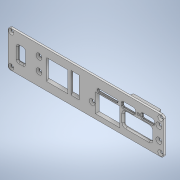
# Autodesk Inventor part: back_panel
Saved by Autodesk Inventor 2021 (Build 250183000, 183)
## iProperties
Created: 2026-03-01
Part Number: back_panel
Material: Generic
Document SubType Name: Modeling
Designer: Toby
Density: 1 g/cm^3
Appearance: Default
Author: Toby
Autodesk Inventor part; units mm, degrees
ref_plane "YZ Plane" through (0, 0, 0) normal (1, 0, 0) x (0, 1, 0)
ref_plane "XZ Plane" through (0, 0, 0) normal (0, 1, 0) x (-1, 0, 0)
ref_plane "XY Plane" through (0, 0, 0) normal (0, 0, 1) x (1, 0, 0)
sketch "Sketch1" plane through (0, 0, 0) normal (0, 0, 1) x (1, 0, 0)
  line L0 (-59.9, 14.1) -> (60.3, 14.1)
  line L1 (60.3, 14.1) -> (60.3, -14.1)
  line L2 (60.3, -14.1) -> (-59.9, -14.1)
  line L3 (-59.9, -14.1) -> (-59.9, 14.1)
  point P0 (0, 0)
  dimension "d0" = 120.2
  dimension "d1" = 28.2
  dimension "d2" = 59.9
  dimension "d3" = 14.1
  constraints: 8 end point, 2 parallel, 1 horizontal, 1 perpendicular
  measures "d0" distance of L0.start L0.end
  measures "d1" distance of L2.end L0.start
  measures "d2" distance from line of point (0, 0) L3
  measures "d3" distance from line of point (0, 0) L0
extrude "Extrusion1" add sketch "Sketch1" along normal blind 1.5
fillet "Fillet1" radius 2 4 edges at (-59.9, 14.1, 0.75) (60.3, 14.1, 0.75) (60.3, -14.1, 0.75) (-59.9, -14.1, 0.75)
sketch "Sketch2" plane through (0, 0, 1.5) normal (0, 0, 1) x (1, 0, 0)
  line L0 (-59.9, 12.1) -> (-59.9, -12.1) projected
  line L1 (58.3, 14.1) -> (-57.9, 14.1) projected
  line L2 (-57.9, -14.1) -> (58.3, -14.1) projected
  line L3 (60.3, -12.1) -> (60.3, 12.1) projected
  point P0 (0, 0)
  point P1 (-57.5, 11.7)
  point P2 (-57.5, -11.7)
  point P3 (57.9, 11.7)
  point P4 (57.9, -11.7)
  dimension "d7" = 2.4
  dimension "d8" = 2.4
  dimension "d9" = 2.4
  dimension "d10" = 2.4
  dimension "d11" = 2.4
  dimension "d12" = 2.4
  dimension "d13" = 2.4
  dimension "d14" = 2.4
  measures "d7" distance from line of L0 point (-57.5, 11.7)
  measures "d8" distance from line of L1 point (-57.5, 11.7)
  measures "d9" distance from line of L2 point (-57.5, -11.7)
  measures "d10" distance from line of L0 point (-57.5, -11.7)
  measures "d11" distance from line of L1 point (57.9, 11.7)
  measures "d12" distance from line of L3 point (57.9, 11.7)
  measures "d13" distance from line of L2 point (57.9, -11.7)
  measures "d14" distance from line of L3 point (57.9, -11.7)
hole "Hole1" at (-57.5, 11.7, 1.5) at (-57.5, -11.7, 1.5) at (57.9, 11.7, 1.5) at (57.9, -11.7, 1.5) direction (0, 0, -1) diameter 2 depth 4 tip angle 118 countersink diameter 4 countersink angle 90
sketch "Sketch3" plane through (0, 0, 1.5) normal (0, 0, 1) x (1, 0, 0)
  circle A0 centre (-57.5, -11.7) radius 1 projected
  circle A1 centre (-57.5, 11.7) radius 1 projected
  line L0 (-55.9, 14.1) -> (60.3, 14.1)
  line L1 (60.3, 14.1) -> (60.3, -14)
  line L2 (60.3, -14) -> (-55.9, -14)
  line L3 (-55.9, -14) -> (-55.9, 14.1)
  line L4 (-59.9, 12.1) -> (-59.9, -12.1) projected
  line L5 (-57.9, -14.1) -> (58.3, -14.1) projected
  line L6 (58.3, 14.1) -> (-57.9, 14.1) projected
  line L7 (60.3, -12.1) -> (60.3, 12.1) projected
  line L8 (-52.5, 5.1) -> (-47.3, 5.1)
  line L9 (-47.3, 5.1) -> (-47.3, -5.6)
  line L10 (-47.3, -5.6) -> (-52.5, -5.6)
  line L11 (-52.5, -5.6) -> (-52.5, 5.1)
  circle A2 centre (-35.9, 6) radius 1
  circle A3 centre (-35.9, -4) radius 1
  circle A4 centre (5.1, -4) radius 1
  circle A5 centre (56.6, -4) radius 1
  circle A6 centre (56.6, 6) radius 1
  line L12 (-30, 6.7) -> (-13.7, 6.7)
  line L13 (-13.7, 6.7) -> (-13.7, -6.3)
  line L14 (-13.7, -6.3) -> (-30, -6.3)
  line L15 (-30, -6.3) -> (-30, 6.7)
  line L16 (9.1, 4) -> (25.1, 4)
  line L17 (25.1, 4) -> (25.1, -9)
  line L18 (25.1, -9) -> (9.1, -9)
  line L19 (9.1, -9) -> (9.1, 4)
  line L20 (29.1, 2) -> (51.1, 2)
  line L21 (51.1, 2) -> (51.1, -8)
  line L22 (51.1, -8) -> (29.1, -8)
  line L23 (29.1, -8) -> (29.1, 2)
  line L24 (28.1, 7.9) -> (38, 7.9)
  line L25 (38, 7.9) -> (38, 4.2)
  line L26 (38, 4.2) -> (28.1, 4.2)
  line L27 (28.1, 4.2) -> (28.1, 7.9)
  line L28 (43.3, 7.9) -> (52.8, 7.9)
  line L29 (52.8, 7.9) -> (52.8, 4.2)
  line L30 (52.8, 4.2) -> (43.3, 4.2)
  line L31 (43.3, 4.2) -> (43.3, 7.9)
  line L32 (-11.2, 7.5) -> (-4.9, 7.5)
  line L33 (-4.9, 7.5) -> (-4.9, -6)
  line L34 (-4.9, -6) -> (-11.2, -6)
  line L35 (-11.2, -6) -> (-11.2, 7.5)
  line L36 (9.1, 5) -> (25.1, 5)
  line L37 (25.1, 5) -> (25.1, 7.5)
  line L38 (25.1, 7.5) -> (9.1, 7.5)
  line L39 (9.1, 7.5) -> (9.1, 5)
  point P0 (0, 0)
  dimension "d22" = 23.4
  dimension "d23" = 4
  dimension "d24" = 0.1
  dimension "d25" = 8.4
  dimension "d26" = 19.1
  dimension "d27" = 3.4
  dimension "d28" = 8.6
  dimension "d31" = 2
  dimension "d32" = 2
  dimension "d35" = 10
  dimension "d36" = 10
  dimension "d37" = 2
  dimension "d38" = 61
  dimension "d39" = 10
  dimension "d40" = 2
  dimension "d41" = 2
  dimension "d42" = 112.5
  dimension "d43" = 112.5
  dimension "d45" = 20
  dimension "d46" = 10
  dimension "d47" = 25.9
  dimension "d48" = 42.2
  dimension "d49" = 7.7
  dimension "d50" = 20.7
  dimension "d51" = 44.7
  dimension "d52" = 51
  dimension "d53" = 21.5
  dimension "d54" = 8
  dimension "d55" = 65
  dimension "d56" = 81
  dimension "d57" = 85
  dimension "d58" = 107
  dimension "d59" = 5
  dimension "d60" = 18
  dimension "d61" = 6
  dimension "d62" = 16
  dimension "d63" = 2.5
  dimension "d64" = 1
  dimension "d65" = 84
  dimension "d66" = 93.9
  dimension "d67" = 99.2
  dimension "d68" = 108.7
  dimension "d69" = 18.2
  dimension "d70" = 22
  dimension "d104" = 20
  dimension "d105" = 20
  constraints: 72 end point, 18 parallel, 9 horizontal, 9 perpendicular, 5 centre point, 4 collinear, 2 point on line
  measures "d22" distance of A0.centre A1.centre
  measures "d23" distance between parallel lines of L4 L3
  measures "d24" distance between parallel lines of L5 L2
  measures "d25" distance between parallel lines of L2 L10
  measures "d26" distance between parallel lines of L2 L8
  measures "d27" distance between parallel lines of L3 L11
  measures "d28" distance between parallel lines of L3 L9
  measures "d31" diameter of A2
  measures "d32" diameter of A3
  measures "d35" distance from line of A3.centre L2
  measures "d36" distance of A3.centre A2.centre
  measures "d37" diameter of A4
  measures "d38" distance from line of L3 A4.centre
  measures "d39" distance from line of L2 A4.centre
  measures "d40" diameter of A5
  measures "d41" diameter of A6
  measures "d42" distance from line of L3 A5.centre
  measures "d43" distance from line of L3 A6.centre
  measures "d45" distance from line of L2 A6.centre
  measures "d46" distance from line of L2 A5.centre
  measures "d47" distance between parallel lines of L3 L15
  measures "d48" distance between parallel lines of L3 L13
  measures "d49" distance between parallel lines of L2 L14
  measures "d50" distance between parallel lines of L2 L12
  measures "d51" distance between parallel lines of L3 L35
  measures "d52" distance between parallel lines of L3 L33
  measures "d53" distance between parallel lines of L2 L32
  measures "d54" distance between parallel lines of L2 L34
  measures "d55" distance between parallel lines of L3 L19
  measures "d56" distance between parallel lines of L3 L17
  measures "d57" distance between parallel lines of L3 L23
  measures "d58" distance between parallel lines of L3 L21
  measures "d59" distance between parallel lines of L2 L18
  measures "d60" distance between parallel lines of L2 L16
  measures "d61" distance between parallel lines of L2 L22
  measures "d62" distance between parallel lines of L2 L20
  measures "d63" distance between parallel lines of L36 L38
  measures "d64" distance between parallel lines of L16 L36
  measures "d65" distance between parallel lines of L3 L27
  measures "d66" distance between parallel lines of L3 L25
  measures "d67" distance between parallel lines of L3 L31
  measures "d68" distance between parallel lines of L3 L29
  measures "d69" distance between parallel lines of L2 L26
  measures "d70" distance between parallel lines of L5 L24
  measures "d104" distance from line of L3 A2.centre
  measures "d105" distance from line of L3 A3.centre
extrude "Extrusion2" cut sketch "Sketch3" against normal blind 1.5 contours L8 L9 L10 L11 | A2 | A3 | A4 | A5 | A6 | L12 L13 L14 L15 | L16 L17 L18 L19 | L20 L21 L22 L23 | L24 L25 L26 L27 | L28 L29 L30 L31 | L32 L33 L34 L35 | L39 L38 L37 L36
fillet "Fillet3" radius 1 8 edges at (28.1, 7.9, 0.75) (28.1, 4.2, 0.75) (38, 7.9, 0.75) (38, 4.2, 0.75) (43.3, 7.9, 0.75) (43.3, 4.2, 0.75) (52.8, 7.9, 0.75) (52.8, 4.2, 0.75)
fillet "Fillet4" radius 2 4 edges at (29.1, 2, 0.75) (29.1, -8, 0.75) (51.1, -8, 0.75) (51.1, 2, 0.75)
chamfer "Chamfer1" distance 1 angle 45 8 edges at (40.1, 2, 1.5) (50.5142, 1.4142, 1.5) (51.1, -3, 1.5) (50.5142, -7.4142, 1.5) (40.1, -8, 1.5) (29.6858, -7.4142, 1.5) (29.1, -3, 1.5) (29.6858, 1.4142, 1.5)
fillet "Fillet5" radius 1 4 edges at (-52.5, 5.1, 0.75) (-47.3, 5.1, 0.75) (-52.5, -5.6, 0.75) (-47.3, -5.6, 0.75)
chamfer "Chamfer2" distance 0.6 angle 45 16 edges at (33.05, 7.9, 1.5) (37.7071, 7.6071, 1.5) (38, 6.05, 1.5) (37.7071, 4.4929, 1.5) (33.05, 4.2, 1.5) (28.3929, 4.4929, 1.5) (28.1, 6.05, 1.5) (28.3929, 7.6071, 1.5) (48.05, 7.9, 1.5) (52.5071, 7.6071, 1.5) (52.8, 6.05, 1.5) (52.5071, 4.4929, 1.5) (48.05, 4.2, 1.5) (43.5929, 4.4929, 1.5) (43.3, 6.05, 1.5) (43.5929, 7.6071, 1.5)
chamfer "Chamfer4" distance 1 angle 45 8 edges at (-49.9, 5.1, 1.5) (-47.5929, 4.8071, 1.5) (-47.3, -0.25, 1.5) (-47.5929, -5.3071, 1.5) (-49.9, -5.6, 1.5) (-52.2071, -5.3071, 1.5) (-52.5, -0.25, 1.5) (-52.2071, 4.8071, 1.5)
fillet "Fillet6" radius 1 4 edges at (9.1, 7.5, 0.75) (9.1, 5, 0.75) (25.1, 7.5, 0.75) (25.1, 5, 0.75)
sketch "Sketch4" plane through (0, 0, 1.5) normal (0, 0, 1) x (1, 0, 0)
  line L0 (43.3, 5.2) -> (43.3, 6.9) projected
  line L1 (38, 6.9) -> (38, 5.2) projected
  line L2 (44.3, 3.6) -> (51.8, 3.6) projected
  circle A0 centre (40.8, 5.8) radius 1
  point P0 (0, 0)
  dimension "d88" = 5.3
  dimension "d89" = 2.5
  dimension "d90" = 2.2
  dimension "d91" = 2
  constraints: 1 centre point, 1 coincident
  measures "d88" distance between parallel lines of L0 L1
  measures "d89" distance from line of L0 point (40.8, 5.8)
  measures "d90" distance from line of L2 point (40.8, 5.8)
  measures "d91" diameter of A0
extrude "Extrusion3" cut sketch "Sketch4" against normal blind 1.5
sketch "Sketch5" plane through (0, 0, 0) normal (0, 0, -1) x (-1, 0, 0)
  line L0 (-52.3, 11.1) -> (-30.3, 11.1)
  line L1 (-30.3, 11.1) -> (-30.3, 9.1)
  line L2 (-30.3, 9.1) -> (-52.3, 9.1)
  line L3 (-52.3, 9.1) -> (-52.3, 11.1)
  line L4 (57.9, -14.1) -> (-58.3, -14.1) projected
  line L5 (-60.3, -12.1) -> (-60.3, 12.1) projected
  line L6 (-58.3, 14.1) -> (57.9, 14.1) projected
  point P0 (0, 0)
  dimension "d94" = 23.2
  dimension "d95" = 8
  dimension "d96" = 30
  dimension "d97" = 2
  dimension "d109" = 5
  constraints: 8 end point, 2 parallel, 1 horizontal, 1 perpendicular
  measures "d94" distance between parallel lines of L4 L2
  measures "d95" distance between parallel lines of L5 L3
  measures "d96" distance between parallel lines of L5 L1
  measures "d97" distance between parallel lines of L2 L0
  measures "d109" distance between parallel lines of L2 L6
extrude "Extrusion4" add sketch "Sketch5" along normal blind 5
chamfer "Chamfer5" distance 2 angle 45 1 edges at (41.3, 11.1, 0)
fillet "Fillet7" radius 1 2 edges at (52.3, 10.1, -5) (30.3, 10.1, -5)
chamfer "Chamfer6" distance 1.5 angle 45 3 edges at (9.1, -2.5, 1.5) (25.1, -2.5, 1.5) (17.1, -9, 1.5)
chamfer "Chamfer7" distance 1.5 angle 45 4 edges at (-21.85, -6.3, 1.5) (-21.85, 6.7, 1.5) (-8.05, 7.5, 1.5) (-8.05, -6, 1.5)
sketch "Sketch6" plane through (0, 0, 1.5) normal (0, 0, 1) x (1, 0, 0)
  circle A0 centre (-35.9, 6) radius 1 projected
  circle A1 centre (-35.9, -4) radius 1 projected
  circle A2 centre (5.1, -4) radius 1 projected
  circle A3 centre (56.6, -4) radius 1 projected
  circle A4 centre (56.6, 6) radius 1 projected
  point P0 (0, 0)
  constraints: 5 coincident
hole "Hole2" at (-35.9, 6, 1.5) at (-35.9, -4, 1.5) at (5.1, -4, 1.5) at (56.6, -4, 1.5) at (56.6, 6, 1.5) direction (0, 0, -1) diameter 2 depth 4 tip angle 118 countersink diameter 4.5 countersink angle 90
body "Solid1"
